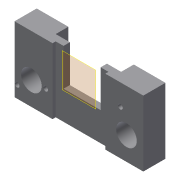
# Autodesk Inventor part: 20_Adapter_Bluray_KES400_Lens_Thorlabs_v2
Saved by Autodesk Inventor 2019 (Build 230136000, 136)
## iProperties
Created: 2018-09-25
Part Number: 20_Adapter_Bluray_KES400_Lens_Thorlabs_v2
Material: Generic
Document SubType Name: Modeling
Designer: diederichbenedict
Density: 1 g/cm^3
Appearance: Default
Author: diederichbenedict
Autodesk Inventor part; units mm, degrees
ref_plane "YZ Plane" through (0, 0, 0) normal (1, 0, 0) x (0, 1, 0)
ref_plane "XZ Plane" through (0, 0, 0) normal (0, 1, 0) x (-1, 0, 0)
ref_plane "XY Plane" through (0, 0, 0) normal (0, 0, 1) x (1, 0, 0)
ref_plane "Work Plane1" through (0, 37.4307, 11.591) normal (0, 0, 1) x (1, 0, 0)
sketch "Sketch1" plane through (0, 37.4307, 11.591) normal (0, 0, 1) x (1, 0, 0)
  circle A0 centre (0, 0) radius 1.2261 construction
  line L0 (4.85, 4.85) -> (-4.85, 4.85) construction
  line L1 (-4.85, 4.85) -> (-4.85, -4.85) construction
  line L2 (-4.85, -4.85) -> (4.85, -4.85) construction
  line L3 (4.85, -4.85) -> (4.85, 4.85) construction
  line L4 (5.85, 5.85) -> (-5.85, 5.85)
  line L5 (-5.85, 5.85) -> (-5.85, -5.85)
  line L6 (-5.85, -5.85) -> (5.85, -5.85)
  line L7 (5.85, -5.85) -> (5.85, 5.85)
  line L8 (20.32, 25.4487) -> (20.32, -10.6193) projected
  line L9 (-20.32, -10.6193) -> (-20.32, 25.4487) projected
  line L10 (5.85, 5.85) -> (20.32, 5.85)
  line L11 (20.32, 5.85) -> (20.32, -5.85)
  line L12 (20.32, -5.85) -> (5.85, -5.85)
  line L13 (5.85, -5.85) -> (5.85, 5.85)
  line L14 (-5.85, 5.85) -> (-20.32, 5.85)
  line L15 (-20.32, 5.85) -> (-20.32, -5.85)
  line L16 (-20.32, -5.85) -> (-5.85, -5.85)
  line L17 (-5.85, -5.85) -> (-5.85, 5.85)
  line L18 (18.034, -12.9053) -> (-18.034, -12.9053) projected
  line L19 (20.32, -5.85) -> (-20.32, -5.85)
  line L20 (-20.32, -5.85) -> (-20.32, -12.9053)
  line L21 (-20.32, -12.9053) -> (20.32, -12.9053)
  line L22 (20.32, -12.9053) -> (20.32, -5.85)
  point P0 (0, -37.4307)
  dimension "d0" = 1
  constraints: 32 end point, 6 parallel, 3 horizontal, 3 perpendicular, 3 point on line, 3 other
  measures "d0" distance between parallel lines of L3 L7
ref_plane "Work Plane2" through (-20.066, 24.7794, 0) normal (0, 0, 1) x (1, 0, 0)
extrude "Extrusion1" add sketch "Sketch1" against normal blind 3 contours L10 L8 L12 L7 | L5 L16 L9 L14 | L12 L8 L22 L21 L18 L20 L9 L16 L6
sketch "Sketch2" plane through (20.32, 24.5254, 11.591) normal (0, 0, -1) x (-1, 0, 0)
  circle A0 centre (35.32, 5.32) radius 3.0099 projected
  circle A1 centre (5.32, 5.32) radius 3.0099 projected
  circle A2 centre (35.32, 5.32) radius 3.2639 projected
  circle A3 centre (5.32, 5.32) radius 3.2639 projected
extrude "Extrusion2" cut sketch "Sketch2" along normal through all contours A0 | A1 | A2 | A3
sketch "Sketch9" plane through (0, 37.4307, 8.591) normal (0, 0, -1) x (-1, 0, 0)
  line L0 (5.85, -5.85) -> (-5.85, -5.85) projected
  circle A0 centre (-15, -7.5852) radius 3.2639 projected
  line L1 (-20.32, 5.85) -> (-20.32, -12.9053) projected
  line L2 (-20.32, -12.9053) -> (20.32, -12.9053) projected
  line L3 (20.32, -12.9053) -> (20.32, 5.85) projected
  circle A1 centre (15, -7.5852) radius 3.2639 projected
  line L4 (-5.85, 5.85) -> (-20.32, 5.85) projected
  line L5 (20.32, 5.85) -> (5.85, 5.85) projected
  line L6 (5.85, 5.85) -> (5.85, -5.85) projected
  line L7 (-5.85, -5.85) -> (-5.85, 5.85) projected
  line L8 (20.32, 5.85) -> (20.32, -12.9053) projected
  line L9 (20.32, 5.85) -> (5.85, 5.85) projected
  line L10 (20.32, -12.9053) -> (10.32, -12.9053)
  line L11 (10.32, -12.9053) -> (10.32, 5.85)
  line L12 (10.32, 5.85) -> (20.32, 5.85)
  line L13 (20.32, 5.85) -> (20.32, -12.9053)
  line L14 (-20.32, -12.9053) -> (-10.32, -12.9053)
  line L15 (-10.32, -12.9053) -> (-10.32, 5.85)
  line L16 (-10.32, 5.85) -> (-20.32, 5.85)
  line L17 (-20.32, 5.85) -> (-20.32, -12.9053)
  point P0 (0, -37.4307)
  dimension "d36" = 10
  dimension "d37" = 10
  constraints: 16 end point, 4 parallel, 2 horizontal, 2 perpendicular, 2 point on line
  measures "d36" distance of L11.end L12.end
  measures "d37" distance of L16.end L15.end
extrude "Extrusion9" add sketch "Sketch9" along normal blind 4 contours L5 L3 L2 L11 | L15 L2 L1 L4
sketch "Sketch10" plane through (-20.32, 24.5254, 11.591) normal (0, -1, 0) x (1, 0, 0)
  line L0 (0, 0) -> (40.64, 0) projected
  line L1 (0, 0) -> (0, -7) projected
  line L2 (10, -7) -> (0, -7) projected
  line L3 (10, -3) -> (10, -7) projected
  line L4 (30.64, -3) -> (10, -3) projected
  line L5 (30.64, -3) -> (30.64, -7) projected
  line L6 (40.64, -7) -> (30.64, -7) projected
  line L7 (40.64, 0) -> (40.64, -7) projected
  point P0 (20.32, -11.591)
extrude "Extrusion10" add sketch "Sketch10" along normal blind 2
sketch "Sketch11" plane through (0, 37.4307, 11.591) normal (0, 0, 1) x (1, 0, 0)
  circle A0 centre (-40.9999, 4.4119) radius 1 projected
  circle A1 centre (-19.4999, -11.0881) radius 1 projected
  circle A2 centre (-12.9999, 9.4119) radius 1 projected
  circle A3 centre (-10.5, -7.6734) radius 1 projected
  circle A4 centre (-17, 12.8266) radius 1 projected
  circle A5 centre (11, 7.8266) radius 1 projected
  point P0 (6.3071, -26.4348)
  point P1 (13.066, -0.8064)
hole "Hole1" at (13.066, 36.6243, 11.591) at (6.3071, 10.9959, 11.591) at (-40.9999, 41.8426, 11.591) at (-19.4999, 26.3426, 11.591) at (-10.5, 29.7573, 11.591) direction (0, 0, -1) diameter 1.5 end through all
sketch "Sketch12" plane through (-20.32, 22.5254, 11.591) normal (0, -1, 0) x (1, 0, 0)
  line L0 (40.64, 0) -> (0, 0) projected
  line L1 (0, 0) -> (0, -7) projected
  line L2 (0, -7) -> (10, -7) projected
  line L3 (10, -7) -> (10, -3) projected
  line L4 (10, -3) -> (30.64, -3) projected
  line L5 (30.64, -3) -> (30.64, -7) projected
  line L6 (30.64, -7) -> (40.64, -7) projected
  line L7 (40.64, -7) -> (40.64, 0) projected
  line L8 (40.64, 0) -> (26.17, 0) projected
  line L9 (28.64, 0) -> (12, 0)
  line L10 (12, 0) -> (12, -1)
  line L11 (12, -1) -> (28.64, -1)
  line L12 (28.64, -1) -> (28.64, 0)
  point P0 (20.32, -11.591)
  dimension "d49" = 1
  dimension "d52" = 2
  dimension "d53" = 2
  constraints: 8 end point, 2 parallel, 1 horizontal, 1 perpendicular, 1 point on line
  measures "d49" distance of L10.end L9.end
  measures "d52" distance between parallel lines of L10 L3
  measures "d53" distance between parallel lines of L12 L5
extrude "Extrusion11" cut sketch "Sketch12" against normal through all contours L12 L11 L10 L0
body "Solid1"
